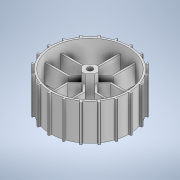
# Autodesk Inventor part: Reifen_v2
Saved by Autodesk Inventor 2021 (Build 250183000, 183)
## iProperties
Created: 2021-01-03
Part Number: Reifen_v2
Material: Generisch
Document SubType Name: Modeling
Designer: Ctroi
Density: 1 g/cm^3
Appearance: Vorgabe
Author: Ctroi
## iProperties of the stored document _3D-Druck.ipt
Created: 2021-01-03
Part Number: _3D-Druck
Material: Generisch
Document SubType Name: Modeling
Designer: Ctroi
Density: 1 g/cm^3
Appearance: Vorgabe
Author: Ctroi
Autodesk Inventor part; units mm, degrees
ref_plane "YZ Plane" through (0, 0, 0) normal (1, 0, 0) x (0, 1, 0)
ref_plane "XZ Plane" through (0, 0, 0) normal (0, 1, 0) x (-1, 0, 0)
ref_plane "XY Plane" through (0, 0, 0) normal (0, 0, 1) x (1, 0, 0)
sketch "Grundskizze" plane through (0, 0, 0) normal (0, 1, 0) x (-1, 0, 0)
  circle A0 centre (0, 0) radius 65
  circle A1 centre (0, 0) radius 62
  circle A2 centre (0, 0) radius 4.5
  line L0 (11, -3.1421) -> (3.1421, -11)
  line L1 (-3.1421, -11) -> (-11, -3.1421)
  line L2 (-11, 3.1421) -> (-3.1421, 11)
  line L3 (3.1421, 11) -> (11, 3.1421)
  line L4 (0, -91) -> (0, 91) projected
  line L5 (91, 0) -> (-91, 0) projected
  line L6 (3.1421, -11) -> (-3.1421, -11)
  line L7 (-11, -3.1421) -> (-11, 3.1421)
  line L8 (-3.1421, 11) -> (3.1421, 11)
  line L9 (11, 3.1421) -> (11, -3.1421)
  line L10 (3.1421, -11) -> (13.7487, -21.6066)
  line L11 (3.1421, -11) -> (18.1421, -11) construction
  line L12 (13.7487, -21.6066) -> (13.7487, -60.4564)
  line L13 (-3.1421, -11) -> (-15.1738, -23.0317)
  line L14 (-3.1421, -11) -> (13.8732, -11) construction
  line L15 (-15.1738, -23.0317) -> (-15.1738, -60.1145)
  line L16 (10.7487, -44.9441) -> (10.7487, -22.8492)
  line L17 (10.7487, -22.8492) -> (1.0208, -13.1213)
  line L18 (-12.1738, -44.9441) -> (-12.1738, -24.2743)
  line L19 (-12.1738, -24.2743) -> (-1.0208, -13.1213)
  line L20 (1.0208, -13.1213) -> (-1.0208, -13.1213)
  line L21 (10.7487, -44.9441) -> (10.7487, -61.0612)
  line L22 (-12.1738, -44.9441) -> (-12.1738, -60.7931)
  line L23 (23.0317, -15.1738) -> (60.1145, -15.1738)
  line L24 (44.9441, -12.1738) -> (60.7931, -12.1738)
  line L25 (44.9441, -12.1738) -> (24.2743, -12.1738)
  line L26 (24.2743, -12.1738) -> (13.1213, -1.0208)
  line L27 (11, -3.1421) -> (23.0317, -15.1738)
  line L28 (22.8492, 10.7487) -> (13.1213, 1.0208)
  line L29 (13.1213, 1.0208) -> (13.1213, -1.0208)
  line L30 (11, 3.1421) -> (21.6066, 13.7487)
  line L31 (44.9441, 10.7487) -> (22.8492, 10.7487)
  line L32 (21.6066, 13.7487) -> (60.4564, 13.7487)
  line L33 (44.9441, 10.7487) -> (61.0612, 10.7487)
  line L34 (15.1738, 23.0317) -> (15.1738, 60.1145)
  line L35 (12.1738, 44.9441) -> (12.1738, 60.7931)
  line L36 (12.1738, 44.9441) -> (12.1738, 24.2743)
  line L37 (12.1738, 24.2743) -> (1.0208, 13.1213)
  line L38 (3.1421, 11) -> (15.1738, 23.0317)
  line L39 (-10.7487, 22.8492) -> (-1.0208, 13.1213)
  line L40 (-1.0208, 13.1213) -> (1.0208, 13.1213)
  line L41 (-3.1421, 11) -> (-13.7487, 21.6066)
  line L42 (-10.7487, 44.9441) -> (-10.7487, 22.8492)
  line L43 (-13.7487, 21.6066) -> (-13.7487, 60.4564)
  line L44 (-10.7487, 44.9441) -> (-10.7487, 61.0612)
  line L45 (-23.0317, 15.1738) -> (-60.1145, 15.1738)
  line L46 (-44.9441, 12.1738) -> (-60.7931, 12.1738)
  line L47 (-44.9441, 12.1738) -> (-24.2743, 12.1738)
  line L48 (-24.2743, 12.1738) -> (-13.1213, 1.0208)
  line L49 (-11, 3.1421) -> (-23.0317, 15.1738)
  line L50 (-22.8492, -10.7487) -> (-13.1213, -1.0208)
  line L51 (-13.1213, -1.0208) -> (-13.1213, 1.0208)
  line L52 (-11, -3.1421) -> (-21.6066, -13.7487)
  line L53 (-44.9441, -10.7487) -> (-22.8492, -10.7487)
  line L54 (-21.6066, -13.7487) -> (-60.4564, -13.7487)
  line L55 (-44.9441, -10.7487) -> (-61.0612, -10.7487)
  point P0 (0, -11)
  point P1 (-60.1145, 15.1738)
  point P2 (-60.7931, 12.1738)
  point P3 (-60.4564, -13.7487)
  point P4 (60.1145, -15.1738)
  point P5 (61.0612, 10.7487)
  point P6 (60.4564, 13.7487)
  dimension "d0" = 130
  dimension "d1" = 3
  dimension "d2" = 9
  dimension "d7" = 15
  dimension "d8" = 45
  dimension "d10" = 135
  dimension "d11" = 3
  dimension "d12" = 3
  dimension "d52" = 360
  constraints: 108 end point, 6 vertical, 5 horizontal, 4 parallel, 4 point on circle, 3 centre point, 2 coincident, 2 equal length, 2 perpendicular, 1 midpoint, 110 other
  measures "d0" diameter of A0
  measures "d1" radial gap between concentric circles of A0 A1
  measures "d2" diameter of A2
  measures "d7" distance of L0.end L10.end
  measures "d8" angle of L10 L11
  measures "d10" angle of L13 L14
  measures "d11" distance between parallel lines of L12 L16
  measures "d12" distance between parallel lines of L15 L18
extrude "Außenrahmen" add sketch "Grundskizze" along normal blind 45 and the other way blind 15 contours L5 A1 L4 A0 | A0 L4 A1 L5 | L4 A1 L5 A0 | A0 L5 A1 L4
extrude "Radnabe" add sketch "Grundskizze" along normal blind 45 contours L9 L0 L6 L4 A2 L5 | L5 A2 L4 L8 L3 L9 | L4 A2 L5 L7 L2 L8 | L6 L1 L7 L5 A2 L4
sketch "Profilskizze" plane through (0, 45, 0) normal (0, 1, 0) x (1, 0, 0)
  circle A0 centre (0, 0) radius 65 projected
  circle A1 centre (0, 0) radius 65 projected
  line L0 (1.5, 64.9827) -> (1.5, 68.5)
  line L1 (1, 69) -> (-1, 69)
  line L2 (-1.5, 68.5) -> (-1.5, 64.9827)
  line L3 (0, 94.7134) -> (0, -91.6189) projected
  arc A2 (-1, 69) -> (-1.5, 68.5) centre (-1, 68.5) ccw
  arc A3 (1.5, 68.5) -> (1, 69) centre (1, 68.5) ccw
  point P0 (1.5, 69)
  point P1 (-1.5, 69)
  dimension "d58" = 0.5
  dimension "d64" = 4
  dimension "d65" = 3
  constraints: 6 end point, 6 point on circle, 4 point on line, 4 tangent, 2 centre point, 2 parallel, 1 equal radius, 1 other
  measures "d58" radius of A2
  measures "d64" distance edge to line of A0 L1
  measures "d65" distance between parallel lines of L2 L0
extrude "Extrusion6" add sketch "Grundskizze" along normal blind 30 contours L33 L31 L28 L29 L5 L9 L30 L32 A1 | A1 L23 L27 L9 L5 L29 L26 L25 L24 | A1 L34 L38 L8 L4 L40 L37 L36 L35 | L44 L42 L39 L40 L4 L8 L41 L43 A1 | A1 L15 L13 L6 L4 L20 L19 L18 L22 | L21 L16 L17 L20 L4 L6 L10 L12 A1 | A1 L45 L49 L7 L5 L51 L48 L47 L46 | L55 L53 L50 L51 L5 L7 L52 L54 A1
extrude "Profil" add sketch "Profilskizze" against normal blind 60 contours A0 L3 L1 A3 L0 | A0 L2 A2 L1 L3
pattern_circular "Runde Anordnung1" count 20 over 360 about axis through (0, 0, 0) along (0, 1, 0) of "Profil"
